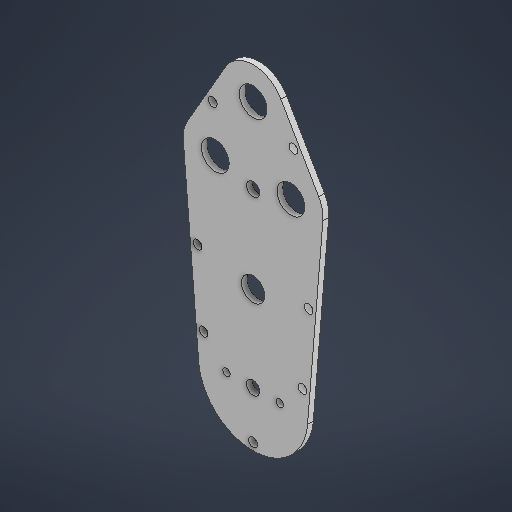
# Autodesk Inventor part: Elo1
Saved by Autodesk Inventor 2025.3 (Build 293356000, 356)
## iProperties
Created: 2025-04-19
Part Number: Elo1
Material: Generic
Document SubType Name: Modeling
Designer: Nelson
Density: 1 g/cm^3
Appearance: Default
Author: Nelson
Autodesk Inventor part; units mm, degrees
ref_plane "YZ Plane" through (0, 0, 0) normal (1, 0, 0) x (0, 1, 0)
ref_plane "XZ Plane" through (0, 0, 0) normal (0, 1, 0) x (-1, 0, 0)
ref_plane "XY Plane" through (0, 0, 0) normal (0, 0, 1) x (1, 0, 0)
ref_plane "Work Plane2" through (0, 0, 0) normal (0, 0, 1) x (1, 0, 0)
sketch "Sketch1" plane through (0, 0, 0) normal (0, 0, 1) x (1, 0, 0)
  line L0 (0, 0) -> (0, 53.385) construction
  circle A0 centre (0, 53.385) radius 11 construction
  circle A1 centre (0, 53.385) radius 30
  circle A2 centre (0, 83.385) radius 9.5
  line L1 (-16, 83.385) -> (16, 83.385) construction
  circle A3 centre (16, 83.385) radius 1.75
  circle A4 centre (-16, 83.385) radius 1.75
  circle A5 centre (-17.9808, 24.5286) radius 1.75
  circle A6 centre (-25.9808, 38.385) radius 9.5
  circle A7 centre (-33.9808, 52.2414) radius 1.75
  circle A8 centre (33.9808, 52.2414) radius 1.75
  circle A9 centre (25.9808, 38.385) radius 9.5
  circle A10 centre (17.9808, 24.5286) radius 1.75
  circle A11 centre (-25.9808, 38.385) radius 20 construction
  circle A12 centre (25.9808, 38.385) radius 20 construction
  circle A13 centre (0, 83.385) radius 20 construction
  line L2 (0, 53.385) -> (0, 31.385) construction
  circle A14 centre (0, 31.385) radius 4.5
  line L3 (0, 53.385) -> (0, -86.615) construction
  circle A15 centre (0, -86.615) radius 37.5
  line L4 (0, 31.385) -> (0, 39.385)
  circle A16 centre (0, 39.385) radius 1.75
  circle A17 centre (-8, 31.385) radius 1.75
  circle A18 centre (0, 23.385) radius 1.75
  circle A19 centre (8, 31.385) radius 1.75
  circle A20 centre (0, -86.615) radius 4.5
  line L5 (0, -86.615) -> (0, -119.115)
  circle A21 centre (0, -119.115) radius 3
  line L6 (0, -86.615) -> (0, -111.615)
  line L7 (0, -86.615) -> (0, -70.365)
  line L8 (0, -70.365) -> (-33.9859, -70.2934)
  circle A22 centre (-33.9859, -70.2934) radius 3
  line L9 (-29.9951, 53.9278) -> (-29.9583, 53.9914)
  circle A23 centre (-25.9808, 38.385) radius 22
  circle A24 centre (0, 83.385) radius 22
  circle A25 centre (25.9808, 38.385) radius 22
  line L10 (-45.0333, 49.385) -> (-19.0526, 94.385)
  line L11 (19.0526, 94.385) -> (45.0333, 49.385)
  line L12 (-37.3702, -89.7323) -> (-47.9046, 36.5562)
  arc A26 (22.9248, 87.6781) -> (-22.9248, 87.6781) centre (0, 53.385) ccw
  arc A27 (-41.1611, 56.0919) -> (41.1611, 56.0919) centre (0, 53.385) ccw
  line L13 (37.3702, -89.7323) -> (47.9046, 36.5562)
  line L14 (-32.0429, 71.885) -> (-27.7128, 69.385)
  circle A28 centre (-27.7128, 69.385) radius 3
  circle A29 centre (33.9859, -70.2934) radius 3
  circle A30 centre (27.7128, 69.385) radius 3
  line L15 (-33.9859, -70.2934) -> (-38.1423, -20.4665)
  line L16 (-43.1027, -21.0096) -> (-38.12, -20.594)
  circle A31 centre (-38.12, -20.594) radius 3
  circle A32 centre (38.12, -20.594) radius 3
  line L17 (0, -86.615) -> (-18.25, -86.615)
  circle A33 centre (-18.25, -86.615) radius 2.5
  circle A34 centre (18.25, -86.615) radius 2.5
  line L18 (0, -86.615) -> (0, -28.03)
  circle A35 centre (0, -28.03) radius 8
  point P0 (-41.0308, 49.1381)
  point P1 (41.0308, 49.1381)
  point P2 (-35.7253, 44.0219)
  point P3 (47.9046, 36.5562)
  dimension "d52" = 75
  dimension "d83" = 44
  dimension "d0" = 53.385
  dimension "d2" = 22
  dimension "d14" = 60
  dimension "d22" = 19
  dimension "d29" = 32
  dimension "d30" = 3.5
  dimension "Fu" = 3.5
  dimension "d34" = 360
  dimension "d43" = 40
  dimension "d46" = 360
  dimension "Lean" = 9
  dimension "d50" = 22
  dimension "d51" = 140
  dimension "d53" = 8
  dimension "d54" = 3.5
  dimension "d57" = 360
  dimension "d61" = 9
  dimension "d62" = 32.5
  dimension "D" = 6
  dimension "d64" = 25
  dimension "d69" = 33.986
  dimension "d70" = 6
  dimension "d81" = 44
  dimension "d82" = 44
  dimension "d84" = 5
  dimension "d85" = 6
  dimension "d88" = 50
  dimension "d89" = 5
  dimension "d90" = 6
  dimension "d91" = 18.25
  dimension "d92" = 5
  dimension "d93" = 58.585
  dimension "d94" = 16
  constraints: 38 end point, 34 centre point, 18 coincident, 12 point on circle, 11 point on line, 8 symmetric about line, 5 tangent, 2 horizontal, 2 midpoint, 2 vertical, 1 perpendicular, 47 other
  measures "d0" distance of L0.start L0.end
  measures "d2" diameter of A0
  measures "d14" diameter of A1
  measures "d22" diameter of A2
  measures "d29" distance of L1.start L1.end
  measures "d30" diameter of A3
  measures "Fu" diameter of A4
  measures "d43" diameter of A11
  measures "Lean" diameter of A14
  measures "d50" distance of L2.start L2.end
  measures "d51" distance of L2.start L3.end
  measures "d53" distance of L4.start L4.end
  measures "d54" diameter of A16
  measures "d61" diameter of A20
  measures "d62" distance of L5.start L5.end
  measures "D" diameter of A21
  measures "d64" distance of L5.start L6.end
  measures "d69" distance of L7.end L8.end
  measures "d70" diameter of A22
  measures "d81" diameter of A23
  measures "d82" diameter of A24
  measures "d84" distance of L14.start L14.end
  measures "d85" diameter of A28
  measures "d88" distance of L15.start L15.end
  measures "d89" distance of L16.start L16.end
  measures "d90" diameter of A31
  measures "d91" distance of L5.start L17.end
  measures "d92" diameter of A33
  measures "d93" distance of L5.start L18.end
  measures "d94" diameter of A35
extrude "Extrusion5" add sketch "Sketch1" along normal blind 4 contours A1 A9 A25 | A1 A25 A27 A9 | A25 A1 A18 A23 A28 A24 A30 | A1 A30 A24 A26 L11 A27 A25 | A27 L11 A25 | A25 A27 | A25 A27 A23 A1 A18 | A25 L13 A15 A29 A22 L15 A31 L16 L12 A23 A27 | A18 A1 | A1 A18 | A24 A1 A2 | A1 A2 A24 A26 | A27 A23 A1 A6 | A23 A27 | A26 A24 L11 | A1 A28 L14 L10 A26 A24 | A15 A22 L8 L18 A29 | A1 A6 A23 | A27 L10 L14 A28 A1 A23 | A23 L10 A27 | A24 A26 | A26 L10 A24 | L12 L16 A31 L15 A22 A15 | A22 A15 L18 L8 | A3 | A4 | A5 | A7 | A8 | A10 | A16 | A17 | A19
equation "\"d30\" = Fu"
equation "\"d70\" = D"
equation "\"d85\" = D"
body "Solid2"
